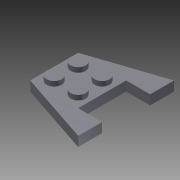
# Autodesk Inventor part: LEGO Brick 4859
Saved by Autodesk Inventor 2011 SP1 (Build 150282100, 282)
## iProperties
Company: Allseas Engineering BV
Created: 2011-09-28
Part Number: LEGO Brick 4859
Cost Center: 0 kg
Material: Steel
Document SubType Name: Modeling
Designer: BvH
Authority: 0 mm^3
Stock Number: =<Filenr>_<Document number>
Density: 7.85 g/cm^3
Act. Code: DW000
SaveDate: 2011-07-28
SaveTime: 18:32
FileName: Standard
TotalMass: 0 kg
TotalVolume: 0 mm^3
Subject: =<Title><TITLE 1_2> <TITLE 2_2>
Author: BvH
Autodesk Inventor part; units mm, degrees
ref_plane "YZ Plane" through (0, 0, 0) normal (1, 0, 0) x (0, 1, 0)
ref_plane "XZ Plane" through (0, 0, 0) normal (0, 1, 0) x (-1, 0, 0)
ref_plane "XY Plane" through (0, 0, 0) normal (0, 0, 1) x (1, 0, 0)
sketch "Sketch1" plane through (0, 0, 0) normal (0, 0, 1) x (1, 0, 0)
  line L0 (-16.8, 0) -> (16.8, 0) construction
  line L1 (0, -22.4) -> (0, 22.4) construction
  line L2 (-12, 16) -> (12, 16)
  line L3 (12, 16) -> (12, -16)
  line L4 (12, -16) -> (-12, -16)
  line L5 (-12, -16) -> (-12, 16)
  line L6 (-8, 4) -> (0, 4) construction
  line L7 (0, 4) -> (0, -4) construction
  line L8 (0, -4) -> (-8, -4) construction
  line L9 (-8, -4) -> (-8, 4) construction
  circle A0 centre (-8, 4) radius 2.5
  circle A1 centre (0, 4) radius 2.5
  circle A2 centre (0, -4) radius 2.5
  circle A3 centre (-8, -4) radius 2.5
  line L10 (12, 8) -> (4, 8)
  line L11 (4, 16) -> (4, -16)
  line L12 (4, -8) -> (12, -8)
  line L13 (12, 16) -> (-12, 8)
  line L14 (12, -16) -> (-12, -8)
  line L15 (8, -12) -> (8, 12) construction
  line L16 (5.5, -14.5) -> (10.5, -14.5)
  line L17 (10.5, -14.5) -> (10.5, -9.5)
  line L18 (10.5, -9.5) -> (5.5, -9.5)
  line L19 (5.5, -9.5) -> (5.5, -14.5)
  line L20 (5.5, 9.5) -> (10.5, 9.5)
  line L21 (10.5, 9.5) -> (10.5, 14.5)
  line L22 (10.5, 14.5) -> (5.5, 14.5)
  line L23 (5.5, 14.5) -> (5.5, 9.5)
  line L24 (5.5, -9.5) -> (10.5, -14.5) construction
  line L25 (5.5, 9.5) -> (10.5, 14.5) construction
  point P0 (12, 0)
  point P1 (0, 16)
  point P2 (0, 0)
  point P3 (4, 0)
  point P4 (8, 0)
  point P5 (8, -8)
  dimension "d0" = 24
  dimension "d1" = 32
  dimension "d2" = 5
  dimension "d3" = 8
  dimension "d4" = 8
  dimension "d5" = 16
  dimension "d10" = 24
  dimension "d11" = 5
  dimension "d14" = 8
  constraints: 50 end point, 15 point on line, 10 midpoint, 8 parallel, 6 horizontal, 4 centre point, 4 coincident, 4 equal length, 4 perpendicular, 3 equal radius, 2 vertical
  measures "d0" distance between parallel lines of L3 L5
  measures "d1" distance between parallel lines of L4 L2
  measures "d2" diameter of A3
  measures "d3" distance between parallel lines of L9 L7
  measures "d4" distance between parallel lines of L3 L11
  measures "d5" distance between parallel lines of L12 L10
  measures "d10" distance of L15.start L15.end
  measures "d11" distance between parallel lines of L17 L19
  measures "d14" distance between parallel lines of L0 L12
extrude "Extrusion1" add sketch "Sketch1" against normal blind 3.2 contours L13 L11 L14 L5 | L3 L10 L11 L13 L23 L20 L21 L22 | L22 L21 L20 L23 L13 | L11 L12 L3 L14 L16 L17 L18 L19 | L19 L18 L17 L16 L14 | A0 | A1 | A2 | A3
extrude "Extrusion2" add sketch "Sketch1" along normal blind 1.6 separate body contours A0 | A1 | A2 | A3
sketch "Sketch3" plane through (0, 0, -3.2) normal (0, 0, -1) x (-1, 0, 0)
  line L0 (-4, 8) -> (-12, 8) projected
  line L1 (-4, -8) -> (-4, 8) projected
  line L2 (-2.5, 6.5) -> (10.5, 6.5)
  line L3 (10.5, 6.5) -> (10.5, -6.5)
  line L4 (10.5, -6.5) -> (-2.5, -6.5)
  line L5 (-2.5, -6.5) -> (-2.5, 6.5)
  circle A0 centre (0, 4) radius 2.5 construction
  circle A1 centre (8, 4) radius 2.5 construction
  circle A2 centre (8, -4) radius 2.5 construction
  circle A3 centre (0, -4) radius 2.5 construction
  circle A4 centre (4, 0) radius 3.1569
  circle A5 centre (4, 0) radius 2.1569
  point P0 (0, 0)
  dimension "d20" = 13
  dimension "d21" = 13
  dimension "d22" = 1.5
  dimension "d23" = 1.5
  dimension "d24" = 1
  constraints: 8 end point, 4 tangent, 2 centre point, 2 parallel, 1 coincident, 1 horizontal, 1 perpendicular
  measures "d20" distance of L3.end L4.end
  measures "d21" distance of L4.end L2.start
  measures "d22" distance between parallel lines of L0 L2
  measures "d23" distance between parallel lines of L1 L5
  measures "d24" radial gap between concentric circles of A5 A4
extrude "Extrusion6" cut sketch "Sketch3" against normal blind 2 bodies 1
sketch "Sketch4" plane through (0, 0, -1.2) normal (0, 0, -1) x (-1, 0, 0)
  line L0 (-12, 16) -> (12, 8) projected
  line L1 (12, 8) -> (12, -8) projected
  line L2 (12, -8) -> (-12, -16) projected
  line L3 (-12, -16) -> (-12, -8) projected
  line L4 (-12, -8) -> (-4, -8) projected
  line L5 (-4, -8) -> (-4, 8) projected
  line L6 (-4, 8) -> (-12, 8) projected
  line L7 (-12, 8) -> (-12, 16) projected
  circle A0 centre (8, -4) radius 2.5 projected
  circle A1 centre (8, 4) radius 2.5 projected
  circle A2 centre (0, 4) radius 2.5 projected
  circle A3 centre (0, -4) radius 2.5 projected
  circle A4 centre (0, 4) radius 1.2
  circle A5 centre (8, 4) radius 1.2
  circle A6 centre (8, -4) radius 1.2
  circle A7 centre (0, -4) radius 1.2
  point P0 (0, 0)
  dimension "d27" = 2.4
  dimension "d28" = 2.4
  dimension "d29" = 2.4
  dimension "d30" = 2.4
  constraints: 4 centre point, 4 coincident
  measures "d27" diameter of A7
  measures "d28" diameter of A6
  measures "d29" diameter of A5
  measures "d30" diameter of A4
extrude "Extrusion7" cut sketch "Sketch4" against normal blind 1 contours A4 | A5 | A6 | A7 bodies 1
equation "\"d28\" = d27"
equation "\"d29\" = d28"
equation "\"d30\" = d29"
body "Solid1"
body "Solid2"
